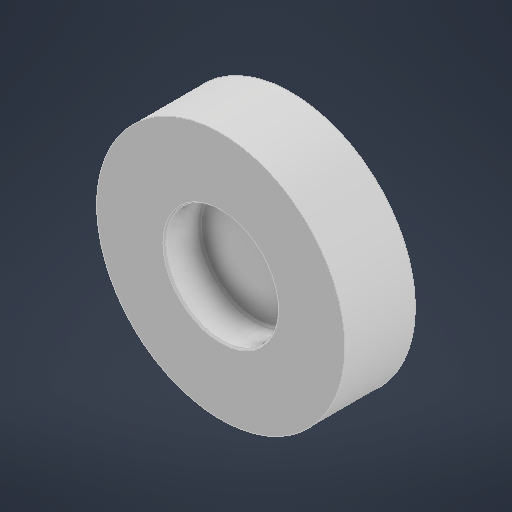
# Autodesk Inventor part: 35mmPetriDishInsert_Diameter16mm_Depth5mm_Biomed
Saved by Autodesk Inventor 2026 (Build 300175050, 175E)
## iProperties
Created: 2024-07-03
Part Number: 35mmPetriDishInsert_Diameter16mm_Depth5mm_Biomed
Material: Kupfer
Document SubType Name: Modeling
Designer: neuhau0004
Density: 8.94 g/cm^3
Appearance: Default
Author: neuhau0004
Autodesk Inventor part; units mm, degrees
ref_plane "YZ Plane" through (0, 0, 0) normal (1, 0, 0) x (0, 1, 0)
ref_plane "XZ Plane" through (0, 0, 0) normal (0, 1, 0) x (-1, 0, 0)
ref_plane "XY Plane" through (0, 0, 0) normal (0, 0, 1) x (1, 0, 0)
sketch "Skizze1" plane through (0, 0, 0) normal (0, 0, 1) x (1, 0, 0)
  circle A0 centre (0, 0) radius 17.6
  circle A1 centre (0, 0) radius 8
  circle A2 centre (0, 0) radius 12
  dimension "d0" = 35.2
  dimension "d1" = 16
  dimension "d2" = 24
  constraints: 3 centre point, 3 coincident
  measures "d0" diameter of A0
  measures "d1" diameter of A1
  measures "d2" diameter of A2
extrude "Extrusion1" add sketch "Skizze1" along normal blind 10 contours A0 | A1 | A2
sketch "Skizze2" plane through (0, 0, 10) normal (0, 0, 1) x (1, 0, 0)
  circle A0 centre (0, 0) radius 8
  circle A1 centre (0, 0) radius 11
  circle A2 centre (0, 0) radius 14
  dimension "d5" = 16
  dimension "d8" = 22
  dimension "d9" = 28
  constraints: 3 centre point, 3 coincident
  measures "d5" diameter of A0
  measures "d8" diameter of A1
  measures "d9" diameter of A2
extrude "Extrusion2" cut sketch "Skizze2" against normal blind 5 contours A0
chamfer "Fase1" distance 0.2 angle 45 1 edges at (-8, 0, 10)
sketch "Skizze3" plane through (0, 0, 10) normal (0, 0, 1) x (1, 0, 0)
  circle A0 centre (0, 0) radius 11.6
  circle A1 centre (0, 0) radius 17.6 projected
  dimension "d13" = 6
  constraints: 1 centre point, 1 coincident, 1 other
  measures "d13" radial gap between concentric circles of A0 A1
feature "Prägen1" [suppressed]
sketch "Skizze4" plane through (0, 0, 0) normal (0, 0, -1) x (-1, 0, 0)
  line L0 (-8.5, 8) -> (8.5, 8) construction
  line L1 (8.5, 8) -> (8.5, -8) construction
  line L2 (8.5, -8) -> (-8.5, -8) construction
  line L3 (-8.5, -8) -> (-8.5, 8) construction
  spline S0 degree 2 poles (-4.8345, 2.8459) (-4.8345, 2.3665) (-5.2231, 1.5951) (-5.5492, 1.3795) knots 0 0 0 1 2 2 2
  spline S1 degree 2 poles (-5.5492, 1.3795) (-5.8158, 1.2122) (-6.3632, 1.0987) (-6.7887, 1.0987) knots 0 0 0 1 2 2 2
  line L4 (-6.7887, 1.0987) -> (-7.5942, 1.0987)
  line L5 (-7.5942, 1.0987) -> (-7.5942, 4.5987)
  line L6 (-7.5942, 4.5987) -> (-6.7972, 4.5987)
  spline S2 degree 2 poles (-6.7972, 4.5987) (-6.3037, 4.5987) (-5.7421, 4.4512) (-5.5436, 4.3208) knots 0 0 0 1 2 2 2
  spline S3 degree 2 poles (-5.5436, 4.3208) (-5.206, 4.0967) (-4.8345, 3.3564) (-4.8345, 2.8459) knots 0 0 0 1 2 2 2
  spline S4 degree 2 poles (-5.3195, 2.8515) (-5.3195, 3.2543) (-5.5861, 3.8244) (-5.8499, 3.9861) knots 0 0 0 1 2 2 2
  spline S5 degree 2 poles (-5.8499, 3.9861) (-6.0371, 4.0967) (-6.4597, 4.196) (-6.7745, 4.196) knots 0 0 0 1 2 2 2
  line L7 (-6.7745, 4.196) -> (-7.1291, 4.196)
  line L8 (-7.1291, 4.196) -> (-7.1291, 1.5015)
  line L9 (-7.1291, 1.5015) -> (-6.7745, 1.5015)
  spline S6 degree 2 poles (-6.7745, 1.5015) (-6.4654, 1.5015) (-5.9974, 1.6007) (-5.8073, 1.734) knots 0 0 0 1 2 2 2
  spline S7 degree 2 poles (-5.8073, 1.734) (-5.5634, 1.8985) (-5.3195, 2.4431) (-5.3195, 2.8515) knots 0 0 0 1 2 2 2
  line L10 (-2.4463, 1.0987) -> (-4.1538, 1.0987)
  line L11 (-4.1538, 1.0987) -> (-4.1538, 1.4561)
  line L12 (-4.1538, 1.4561) -> (-3.5184, 1.4561)
  line L13 (-3.5184, 1.4561) -> (-3.5184, 3.8017)
  line L14 (-3.5184, 3.8017) -> (-4.1538, 3.8017)
  line L15 (-4.1538, 3.8017) -> (-4.1538, 4.1222)
  spline S8 degree 2 poles (-4.1538, 4.1222) (-3.7936, 4.1222) (-3.4532, 4.3264) (-3.4305, 4.6101) knots 0 0 0 1 2 2 2
  line L16 (-3.4305, 4.6101) -> (-3.0675, 4.6101)
  line L17 (-3.0675, 4.6101) -> (-3.0675, 1.4561)
  line L18 (-3.0675, 1.4561) -> (-2.4463, 1.4561)
  line L19 (-2.4463, 1.4561) -> (-2.4463, 1.0987)
  spline S9 degree 2 poles (0.4098, 2.2332) (0.4098, 1.9638) (0.2312, 1.5071) (0.0808, 1.354) knots 0 0 0 1 2 2 2
  spline S10 degree 2 poles (0.0808, 1.354) (-0.0752, 1.1923) (-0.4666, 1.025) (-0.702, 1.025) knots 0 0 0 1 2 2 2
  spline S11 degree 2 poles (-0.702, 1.025) (-0.9374, 1.025) (-1.326, 1.1838) (-1.4735, 1.3426) knots 0 0 0 1 2 2 2
  spline S12 degree 2 poles (-1.4735, 1.3426) (-1.655, 1.5327) (-1.8592, 2.1708) (-1.8592, 2.636) knots 0 0 0 1 2 2 2
  spline S13 degree 2 poles (-1.8592, 2.636) (-1.8592, 3.0926) (-1.672, 3.8272) (-1.4763, 4.0995) knots 0 0 0 1 2 2 2
  spline S14 degree 2 poles (-1.4763, 4.0995) (-1.2863, 4.3661) (-0.685, 4.6639) (-0.2907, 4.6639) knots 0 0 0 1 2 2 2
  spline S15 degree 2 poles (-0.2907, 4.6639) (-0.1744, 4.6639) (0.0298, 4.6413) (0.1064, 4.6157) knots 0 0 0 1 2 2 2
  line L20 (0.1064, 4.6157) -> (0.1064, 4.1648)
  line L21 (0.1064, 4.1648) -> (0.0865, 4.1648)
  spline S16 degree 2 poles (0.0865, 4.1648) (0.0213, 4.1988) (-0.217, 4.2584) (-0.3531, 4.2584) knots 0 0 0 1 2 2 2
  spline S17 degree 2 poles (-0.3531, 4.2584) (-0.7899, 4.2584) (-1.326, 3.6684) (-1.377, 3.0898) knots 0 0 0 1 2 2 2
  spline S18 degree 2 poles (-1.377, 3.0898) (-1.2097, 3.2061) (-0.858, 3.3337) (-0.6481, 3.3337) knots 0 0 0 1 2 2 2
  spline S19 degree 2 poles (-0.6481, 3.3337) (-0.4439, 3.3337) (-0.1376, 3.2515) (0.0298, 3.1267) knots 0 0 0 1 2 2 2
  spline S20 degree 2 poles (0.0298, 3.1267) (0.2226, 2.982) (0.4098, 2.5339) (0.4098, 2.2332) knots 0 0 0 1 2 2 2
  spline S21 degree 2 poles (-0.0667, 2.2134) (-0.0667, 2.4289) (-0.1801, 2.7211) (-0.3049, 2.8232) knots 0 0 0 1 2 2 2
  spline S22 degree 2 poles (-0.3049, 2.8232) (-0.3985, 2.8969) (-0.6311, 2.9451) (-0.753, 2.9451) knots 0 0 0 1 2 2 2
  spline S23 degree 2 poles (-0.753, 2.9451) (-0.9175, 2.9451) (-1.2267, 2.8459) (-1.377, 2.7523) knots 0 0 0 1 2 2 2
  spline S24 degree 2 poles (-1.377, 2.7523) (-1.3799, 2.7012) (-1.3855, 2.6048) (-1.3855, 2.531) knots 0 0 0 1 2 2 2
  spline S25 degree 2 poles (-1.3855, 2.531) (-1.3855, 2.168) (-1.2437, 1.7227) (-1.1359, 1.6064) knots 0 0 0 1 2 2 2
  spline S26 degree 2 poles (-1.1359, 1.6064) (-1.0367, 1.4958) (-0.8211, 1.4079) (-0.6991, 1.4079) knots 0 0 0 1 2 2 2
  spline S27 degree 2 poles (-0.6991, 1.4079) (-0.4155, 1.4079) (-0.0667, 1.8106) (-0.0667, 2.2134) knots 0 0 0 1 2 2 2
  line L22 (4.9678, 1.0987) -> (4.5026, 1.0987)
  line L23 (4.5026, 1.0987) -> (4.5026, 2.8118)
  line L24 (4.5026, 2.8118) -> (2.8916, 2.8118)
  line L25 (2.8916, 2.8118) -> (2.8916, 1.0987)
  line L26 (2.8916, 1.0987) -> (2.4265, 1.0987)
  line L27 (2.4265, 1.0987) -> (2.4265, 4.5987)
  line L28 (2.4265, 4.5987) -> (2.8916, 4.5987)
  line L29 (2.8916, 4.5987) -> (2.8916, 3.2259)
  line L30 (2.8916, 3.2259) -> (4.5026, 3.2259)
  line L31 (4.5026, 3.2259) -> (4.5026, 4.5987)
  line L32 (4.5026, 4.5987) -> (4.9678, 4.5987)
  line L33 (4.9678, 4.5987) -> (4.9678, 1.0987)
  spline S28 degree 2 poles (7.6991, 2.2105) (7.6991, 1.9581) (7.5375, 1.527) (7.39, 1.3682) knots 0 0 0 1 2 2 2
  spline S29 degree 2 poles (7.39, 1.3682) (7.2425, 1.2093) (6.8029, 1.025) (6.5306, 1.025) knots 0 0 0 1 2 2 2
  spline S30 degree 2 poles (6.5306, 1.025) (6.281, 1.025) (5.7932, 1.1356) (5.6145, 1.2235) knots 0 0 0 1 2 2 2
  line L34 (5.6145, 1.2235) -> (5.6145, 1.7199)
  line L35 (5.6145, 1.7199) -> (5.6485, 1.7199)
  spline S31 degree 2 poles (5.6485, 1.7199) (5.7024, 1.6802) (5.9038, 1.578) (6.0257, 1.5327) knots 0 0 0 1 2 2 2
  spline S32 degree 2 poles (6.0257, 1.5327) (6.1647, 1.4844) (6.3944, 1.4306) (6.5391, 1.4306) knots 0 0 0 1 2 2 2
  spline S33 degree 2 poles (6.5391, 1.4306) (6.6809, 1.4306) (6.9475, 1.5327) (7.044, 1.6433) knots 0 0 0 1 2 2 2
  spline S34 degree 2 poles (7.044, 1.6433) (7.1319, 1.7482) (7.2226, 2.0262) (7.2226, 2.2134) knots 0 0 0 1 2 2 2
  spline S35 degree 2 poles (7.2226, 2.2134) (7.2226, 2.4006) (7.1205, 2.6388) (7.0241, 2.7182) knots 0 0 0 1 2 2 2
  spline S36 degree 2 poles (7.0241, 2.7182) (6.9248, 2.8062) (6.6299, 2.8799) (6.4512, 2.8799) knots 0 0 0 1 2 2 2
  spline S37 degree 2 poles (6.4512, 2.8799) (6.2583, 2.8799) (5.8754, 2.8203) (5.7591, 2.7948) knots 0 0 0 1 2 2 2
  line L36 (5.7591, 2.7948) -> (5.7591, 4.5987)
  line L37 (5.7591, 4.5987) -> (7.6793, 4.5987)
  line L38 (7.6793, 4.5987) -> (7.6793, 4.1874)
  line L39 (7.6793, 4.1874) -> (6.2101, 4.1874)
  line L40 (6.2101, 4.1874) -> (6.2101, 3.2543)
  spline S38 degree 2 poles (6.2101, 3.2543) (6.2952, 3.2656) (6.4597, 3.2742) (6.5278, 3.2742) knots 0 0 0 1 2 2 2
  spline S39 degree 2 poles (6.5278, 3.2742) (6.7972, 3.2742) (7.1688, 3.1862) (7.3389, 3.0558) knots 0 0 0 1 2 2 2
  spline S40 degree 2 poles (7.3389, 3.0558) (7.512, 2.9253) (7.6991, 2.5282) (7.6991, 2.2105) knots 0 0 0 1 2 2 2
  line L41 (-4.9096, -4.6639) -> (-6.6171, -4.6639)
  line L42 (-6.6171, -4.6639) -> (-6.6171, -4.3066)
  line L43 (-6.6171, -4.3066) -> (-5.9818, -4.3066)
  line L44 (-5.9818, -4.3066) -> (-5.9818, -1.9609)
  line L45 (-5.9818, -1.9609) -> (-6.6171, -1.9609)
  line L46 (-6.6171, -1.9609) -> (-6.6171, -1.6404)
  spline S41 degree 2 poles (-6.6171, -1.6404) (-6.2569, -1.6404) (-5.9165, -1.4362) (-5.8938, -1.1526) knots 0 0 0 1 2 2 2
  line L47 (-5.8938, -1.1526) -> (-5.5308, -1.1526)
  line L48 (-5.5308, -1.1526) -> (-5.5308, -4.3066)
  line L49 (-5.5308, -4.3066) -> (-4.9096, -4.3066)
  line L50 (-4.9096, -4.3066) -> (-4.9096, -4.6639)
  line L51 (-1.2224, -4.6639) -> (-1.2224, -3.1437)
  spline S42 degree 2 poles (-1.2224, -3.1437) (-1.2224, -2.9622) (-1.2508, -2.653) (-1.2962, -2.5679) knots 0 0 0 1 2 2 2
  spline S43 degree 2 poles (-1.2962, -2.5679) (-1.3416, -2.4743) (-1.5146, -2.3836) (-1.6649, -2.3836) knots 0 0 0 1 2 2 2
  spline S44 degree 2 poles (-1.6649, -2.3836) (-1.8011, -2.3836) (-2.113, -2.5509) (-2.2776, -2.7097) knots 0 0 0 1 2 2 2
  spline S45 degree 2 poles (-2.2776, -2.7097) (-2.2747, -2.7494) (-2.269, -2.8601) (-2.269, -2.9338) knots 0 0 0 1 2 2 2
  line L52 (-2.269, -2.9338) -> (-2.269, -4.6639)
  line L53 (-2.269, -4.6639) -> (-2.7115, -4.6639)
  line L54 (-2.7115, -4.6639) -> (-2.7115, -3.1437)
  spline S46 degree 2 poles (-2.7115, -3.1437) (-2.7115, -2.9622) (-2.7399, -2.653) (-2.7853, -2.5679) knots 0 0 0 1 2 2 2
  spline S47 degree 2 poles (-2.7853, -2.5679) (-2.8306, -2.4743) (-3.0036, -2.3836) (-3.154, -2.3836) knots 0 0 0 1 2 2 2
  spline S48 degree 2 poles (-3.154, -2.3836) (-3.2958, -2.3836) (-3.6106, -2.5622) (-3.7581, -2.7012) knots 0 0 0 1 2 2 2
  line L55 (-3.7581, -2.7012) -> (-3.7581, -4.6639)
  line L56 (-3.7581, -4.6639) -> (-4.2006, -4.6639)
  line L57 (-4.2006, -4.6639) -> (-4.2006, -2.0375)
  line L58 (-4.2006, -2.0375) -> (-3.7581, -2.0375)
  line L59 (-3.7581, -2.0375) -> (-3.7581, -2.3268)
  spline S49 degree 2 poles (-3.7581, -2.3268) (-3.5851, -2.1538) (-3.2447, -1.9638) (-3.0405, -1.9638) knots 0 0 0 1 2 2 2
  spline S50 degree 2 poles (-3.0405, -1.9638) (-2.8079, -1.9638) (-2.4477, -2.1765) (-2.3541, -2.4176) knots 0 0 0 1 2 2 2
  spline S51 degree 2 poles (-2.3541, -2.4176) (-2.1528, -2.1935) (-1.7727, -1.9638) (-1.5515, -1.9638) knots 0 0 0 1 2 2 2
  spline S52 degree 2 poles (-1.5515, -1.9638) (-1.3813, -1.9638) (-1.1033, -2.0687) (-1.0012, -2.1879) knots 0 0 0 1 2 2 2
  spline S53 degree 2 poles (-1.0012, -2.1879) (-0.8963, -2.307) (-0.78, -2.6644) (-0.78, -2.9338) knots 0 0 0 1 2 2 2
  line L60 (-0.78, -2.9338) -> (-0.78, -4.6639)
  line L61 (-0.78, -4.6639) -> (-1.2224, -4.6639)
  line L62 (0.2921, -4.6639) -> (-0.1503, -4.6639)
  line L63 (-0.1503, -4.6639) -> (-0.1503, -1.0079)
  line L64 (-0.1503, -1.0079) -> (0.2921, -1.0079)
  line L65 (0.2921, -1.0079) -> (0.2921, -4.6639)
  line L66 (4.5069, -2.0375) -> (3.517, -4.6639)
  line L67 (3.517, -4.6639) -> (3.1199, -4.6639)
  line L68 (3.1199, -4.6639) -> (2.1386, -2.0375)
  line L69 (2.1386, -2.0375) -> (2.6179, -2.0375)
  line L70 (2.6179, -2.0375) -> (3.3355, -4.0598)
  line L71 (3.3355, -4.0598) -> (4.0474, -2.0375)
  line L72 (4.0474, -2.0375) -> (4.5069, -2.0375)
  line L73 (6.7589, -4.6639) -> (5.0515, -4.6639)
  line L74 (5.0515, -4.6639) -> (5.0515, -4.3066)
  line L75 (5.0515, -4.3066) -> (5.6868, -4.3066)
  line L76 (5.6868, -4.3066) -> (5.6868, -1.9609)
  line L77 (5.6868, -1.9609) -> (5.0515, -1.9609)
  line L78 (5.0515, -1.9609) -> (5.0515, -1.6404)
  spline S54 degree 2 poles (5.0515, -1.6404) (5.4117, -1.6404) (5.752, -1.4362) (5.7747, -1.1526) knots 0 0 0 1 2 2 2
  line L79 (5.7747, -1.1526) -> (6.1378, -1.1526)
  line L80 (6.1378, -1.1526) -> (6.1378, -4.3066)
  line L81 (6.1378, -4.3066) -> (6.7589, -4.3066)
  line L82 (6.7589, -4.3066) -> (6.7589, -4.6639)
  point P0 (0, 0)
  dimension "d16" = 16
  dimension "d17" = 8
  dimension "d18" = 17
  dimension "d19" = 8.5
  constraints: 2 other
  measures "d16" distance between parallel lines of L2 L0
  measures "d17" distance from line of L0 point (0, 0)
  measures "d18" distance of L0.start L0.end
  measures "d19" distance from line of L3 point (0, 0)
emboss "Prägen2" sketch "Skizze4" operation cut depth 0.5 direction (0, 0, 1)
chamfer "Fase2" distance 0.25 angle 45 1 edges at (-8, 0, 5)
